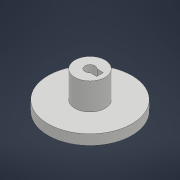
# Autodesk Inventor part: rev_flange_1
Saved by Autodesk Inventor 2022.4 (Build 264492000, 492)
## iProperties
Created: 2016-01-25
Part Number: rev_flange_1
Material: Generic
Document SubType Name: Modeling
Designer: jmacmillan
Density: 1 g/cm^3
Appearance: Default
Mass: 15.0231 g
Surface Area: 62.4678 cm^2
Volume: 15.0231 cm^3
Author: jmacmillan
Autodesk Inventor part; units mm, degrees
ref_plane "YZ Plane" through (0, 0, 0) normal (1, 0, 0) x (0, 1, 0)
ref_plane "XZ Plane" through (0, 0, 0) normal (0, 1, 0) x (-1, 0, 0)
ref_plane "XY Plane" through (0, 0, 0) normal (0, 0, 1) x (1, 0, 0)
sketch "Sketch1" plane through (0, 0, 0) normal (1, 0, 0) x (0, 1, 0)
  line L0 (3, 25) -> (3, 3)
  line L1 (3, 3) -> (25, 3)
  line L2 (25, 3) -> (25, 9)
  line L3 (25, 9) -> (9, 9)
  line L4 (9, 9) -> (9, 25)
  line L5 (9, 25) -> (3, 25)
  line L6 (0, 30) -> (0, -5) projected
  line L7 (-5, 0) -> (30, 0) projected
  point P0 (0, 0)
  dimension "d0" = 6
  dimension "d3" = 22
  dimension "d4" = 3
  dimension "d5" = 3
  constraints: 12 end point, 4 parallel, 3 perpendicular, 1 vertical
  measures "d0" distance of L1.end L2.end
  measures "d3" distance of L0.start L0.end
  measures "d4" distance between parallel lines of L1 L7
  measures "d5" distance between parallel lines of L6 L0
revolve "Revolution1" add sketch "Sketch1" angle 360 about axis through (0, 0, 0) along (0, 0, 1)
sketch "Sketch2" plane through (0, 0, 25) normal (0, 0, 1) x (1, 0, 0)
  circle A0 centre (0, 0) radius 3 projected
  line L0 (2.2361, 2) -> (6, 2)
  line L1 (6, 2) -> (6, -2)
  line L2 (6, -2) -> (2.2361, -2)
  dimension "d7" = 4
  dimension "d9" = 6
  constraints: 6 end point, 2 perpendicular, 2 point on circle, 1 horizontal, 1 parallel
  measures "d7" distance of L0.end L1.end
  measures "d9" distance from line of L1 point (0, 0)
extrude "Extrusion1" cut sketch "Sketch2" against normal blind 16 contours A0 L0 L1 L2
body "Solid1"
